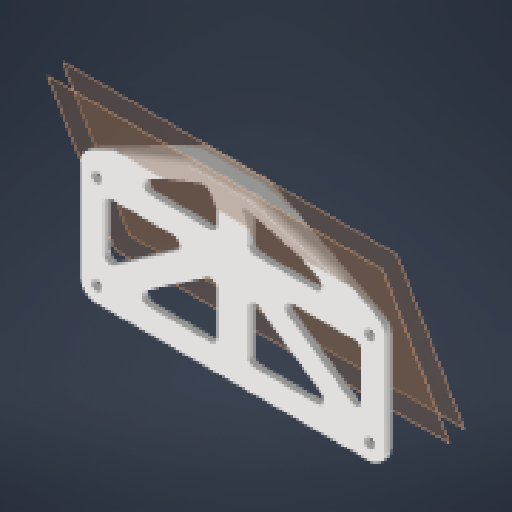
# Autodesk Inventor part: rangoon
Saved by Autodesk Inventor 2025.2 (Build 292293000, 293)
## iProperties
Created: 2025-12-09
Part Number: rangoon
Material: Generic
Document SubType Name: Modeling
Designer: cloudy
Density: 1 g/cm^3
Appearance: Default
Author: cloudy
Autodesk Inventor part; units mm, degrees
ref_plane "YZ Plane" through (0, 0, 0) normal (1, 0, 0) x (0, 1, 0)
ref_plane "XZ Plane" through (0, 0, 0) normal (0, 1, 0) x (-1, 0, 0)
ref_plane "XY Plane" through (0, 0, 0) normal (0, 0, 1) x (1, 0, 0)
sketch "Sketch1" plane through (0, 0, 0) normal (0, 0, 1) x (1, 0, 0)
  circle A0 centre (12.7, -19.05) radius 2.1844 projected
  circle A1 centre (12.7, 19.05) radius 2.1844 projected
  circle A2 centre (-98.425, -19.05) radius 2.1844 projected
  circle A3 centre (-98.425, 19.05) radius 2.1844 projected
  line L0 (19.05, -25.4) -> (-104.775, -25.4)
  line L1 (-104.775, -25.4) -> (-104.775, 25.4)
  line L2 (-104.775, 25.4) -> (19.05, 25.4)
  line L3 (19.05, 25.4) -> (19.05, -25.4)
  line L4 (19.05, -25.4) -> (-104.775, 25.4) construction
  line L5 (-104.775, -25.4) -> (19.05, 25.4) construction
  line L6 (19.05, 25.4) -> (-30.1625, 38.1)
  line L7 (-30.1625, 38.1) -> (-55.5625, 38.1)
  line L8 (-55.5625, 38.1) -> (-104.775, 25.4)
  line L9 (-42.8625, 0) -> (-42.8625, 38.1) construction
  point P0 (0, 0)
  dimension "d0" = 6.35
  dimension "d1" = 6.35
  dimension "d2" = 50.8
  dimension "d3" = 6.35
  dimension "d4" = 12.7
  dimension "d6" = 25.4
  constraints: 20 end point, 3 midpoint, 2 horizontal, 2 parallel, 1 perpendicular, 1 vertical
  measures "d0" distance from line of L3 A0.centre
  measures "d1" distance from line of L1 A2.centre
  measures "d2" distance of L0.end L1.end
  measures "d3" distance from line of L0 A2.centre
  measures "d4" distance between parallel lines of L2 L7
  measures "d6" distance of L6.end L7.end
extrude "Extrusion1" add sketch "Sketch1" along normal blind 2.54
fillet "Fillet1" radius 6.35 6 edges at (19.05, -25.4, 1.27) (19.05, 25.4, 1.27) (-30.1625, 38.1, 1.27) (-55.5625, 38.1, 1.27) (-104.775, 25.4, 1.27) (-104.775, -25.4, 1.27)
sketch "Sketch2" plane through (0, 0, 2.54) normal (0, 0, 1) x (1, 0, 0)
  line L0 (9.525, -11.0599) -> (9.525, 14.2875)
  line L1 (9.525, 14.2875) -> (-27.0917, 14.2875)
  line L2 (-27.0917, 14.2875) -> (9.525, -11.0599)
  line L3 (-12.917, 23.8125) -> (-36.5189, 29.9033)
  line L4 (-36.5189, 29.9033) -> (-36.5189, 23.8125)
  line L5 (-36.5189, 23.8125) -> (-12.917, 23.8125)
  line L6 (-49.2189, 23.8125) -> (-49.2189, 29.9)
  line L7 (-49.2189, 29.9) -> (-72.808, 23.8125)
  line L8 (-72.808, 23.8125) -> (-49.2189, 23.8125)
  line L9 (-0.254, -15.875) -> (-36.5189, 9.2289)
  line L10 (-36.5189, 9.2289) -> (-36.5189, -15.875)
  line L11 (-36.5189, -15.875) -> (-0.254, -15.875)
  line L12 (-49.2189, -15.875) -> (-49.2189, 9.2266)
  line L13 (-49.2189, 9.2266) -> (-85.4731, -15.875)
  line L14 (-85.4731, -15.875) -> (-49.2189, -15.875)
  line L15 (-95.25, -11.0591) -> (-95.25, 14.2875)
  line L16 (-95.25, 14.2875) -> (-58.6421, 14.2875)
  line L17 (-58.6421, 14.2875) -> (-95.25, -11.0591)
  line L18 (-98.425, -25.4) -> (12.7, -25.4) projected
  line L19 (19.05, -19.05) -> (19.05, 20.4807) projected
  arc A0 (-29.3819, 37.8986) -> (-30.9686, 38.1) centre (-30.9686, 31.75) ccw projected
  line L20 (14.2867, 26.6292) -> (-29.3819, 37.8986) projected
  line L21 (-56.3431, 37.8986) -> (-100.0117, 26.6292) projected
  circle A1 centre (12.7, 19.05) radius 2.1844 projected
  line L22 (-104.775, 20.4807) -> (-104.775, -19.05) projected
  circle A2 centre (12.7, -19.05) radius 2.1844 projected
  circle A3 centre (-98.425, -19.05) radius 2.1844 projected
  line L23 (-36.5189, 23.8125) -> (-98.425, -19.05) construction
  line L24 (12.7, -19.05) -> (-49.2189, 23.8125) construction
  point P0 (0, 0)
  point P1 (-30.1689, 38.0494)
  point P2 (-8.7834, 14.2875)
  dimension "d10" = 9.525
  dimension "d11" = 9.525
  dimension "d12" = 12.7
  dimension "d13" = 6.35
  dimension "d14" = 9.525
  dimension "d15" = 9.525
  dimension "d16" = 9.525
  dimension "d17" = 9.525
  dimension "d18" = 4.7625
  dimension "d19" = 9.525
  dimension "d20" = 9.525
  dimension "d21" = 9.525
  dimension "d22" = 4.7625
  dimension "d23" = 4.7625
  constraints: 40 end point, 7 parallel, 6 vertical, 4 collinear, 3 horizontal, 2 perpendicular, 1 midpoint, 1 point on circle
  measures "d10" distance between parallel lines of L18 L11
  measures "d11" distance between parallel lines of L19 L0
  measures "d12" distance between parallel lines of L12 L10
  measures "d13" distance from line of point (-30.169, 38.049) L4
  measures "d14" distance between parallel lines of L16 L8
  measures "d15" distance from line of L5 point (-8.783, 14.287)
  measures "d16" distance between parallel lines of L21 L7
  measures "d17" distance between parallel lines of L20 L3
  measures "d18" distance from line of L5 A1.centre
  measures "d19" distance between parallel lines of L22 L15
  measures "d20" distance between parallel lines of L13 L17
  measures "d21" distance between parallel lines of L2 L9
  measures "d22" distance from line of L24.start L2
  measures "d23" distance from line of L23.end L17
extrude "Extrusion2" cut sketch "Sketch2" against normal through all contours L2 L1 L0 | L5 L4 L3 | L8 L7 L6 | L11 L10 L9 | L14 L13 L12 | L15 L16 L17
fillet "Fillet2" radius 2 18 edges at (-49.2189, 9.2266, 1.27) (-36.5189, 9.2289, 1.27) (-27.0917, 14.2875, 1.27) (-49.2189, 23.8125, 1.27) (-36.5189, 23.8125, 1.27) (-58.6421, 14.2875, 1.27) (-49.2189, 29.9, 1.27) (-36.5189, 29.9033, 1.27) (-72.808, 23.8125, 1.27) (-12.917, 23.8125, 1.27) (9.525, -11.0599, 1.27) (-0.254, -15.875, 1.27) (9.525, 14.2875, 1.27) (-36.5189, -15.875, 1.27) (-49.2189, -15.875, 1.27) (-95.25, 14.2875, 1.27) (-95.25, -11.0591, 1.27) (-85.4731, -15.875, 1.27)
equation "\"d1\" = d0"
equation "\"d3\" = d0"
body "Solid1"
